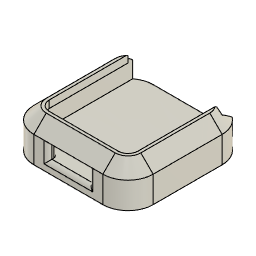
M8Q5883SlideMount (Autodesk Fusion 360 design; units mm, degrees)
Autodesk Fusion 360 part; units mm, degrees
sketch "M8QTop" plane through (0, 0, 0) normal (0, 0, 1) x (1, 0, 0) in component "M8Q"
  line L0 (-7.75, 7.925) -> (7.75, 7.925) construction
  line L1 (7.75, 7.925) -> (7.75, -7.925) construction
  line L2 (7.75, -7.925) -> (-7.75, -7.925) construction
  line L3 (-7.75, -7.925) -> (-7.75, 7.925) construction
  line L4 (0, 7.925) -> (0, -7.925) construction
  line L5 (-7.75, 0) -> (7.75, 0) construction
  line L6 (10, -10) -> (-10, -10) construction
  line L7 (0, 10) -> (0, -10) construction
  line L8 (-10, 10) -> (10, 10) construction
  line L9 (10, 10) -> (10, -10) construction
  line L10 (-10, -10) -> (-10, 10) construction
  line L11 (-10, 0) -> (10, 0) construction
  line L12 (-7, 10) -> (7, 10)
  line L13 (10, 7) -> (10, -7)
  line L14 (7, -10) -> (-7, -10)
  line L15 (-10, -7) -> (-10, 7)
  arc A0 (-7, 10) -> (-10, 7) centre (-7, 7) ccw
  arc A1 (10, 7) -> (7, 10) centre (7, 7) ccw
  arc A2 (7, -10) -> (10, -7) centre (7, -7) ccw
  arc A3 (-10, -7) -> (-7, -10) centre (-7, -7) ccw
  line L16 (-6, 7.925) -> (6, 7.925)
  line L17 (7.75, 6.175) -> (7.75, -6.175)
  line L18 (6, -7.925) -> (-6, -7.925)
  line L19 (-7.75, -6.175) -> (-7.75, 6.175)
  arc A4 (-6, 7.925) -> (-7.75, 6.175) centre (-6, 6.175) ccw
  arc A5 (7.75, 6.175) -> (6, 7.925) centre (6, 6.175) ccw
  arc A6 (6, -7.925) -> (7.75, -6.175) centre (6, -6.175) ccw
  arc A7 (-7.75, -6.175) -> (-6, -7.925) centre (-6, -6.175) ccw
  line L20 (-0.5, 9.134) -> (0.5, 9.134) construction
  line L21 (0.5, 9.134) -> (0, 10) construction
  line L22 (0, 10) -> (-0.5, 9.134) construction
  point P0 (-10, 10)
  point P1 (10, 10)
  point P2 (10, -10)
  point P3 (-7.75, 7.925)
  point P4 (7.75, 7.925)
  point P5 (7.75, -7.925)
  point P6 (0, 9.4226)
  dimension "d16" = 15.5
  dimension "d17" = 15.85
  dimension "d18" = 20
  dimension "d19" = 20
  dimension "d20" = 20
  dimension "d21" = 20
  dimension "d22" = 3
  dimension "d23" = 15.5
  dimension "d24" = 15.85
  dimension "d25" = 1.75
  dimension "d26" = 1
  constraint horizontal L0
  constraint vertical L1
  constraint horizontal L2
  constraint vertical L3
  constraint midpoint L0 L4.start
  constraint midpoint L2 L4.end
  constraint midpoint L3 L5.start
  constraint midpoint L1 L5.end
  constraint horizontal L8
  constraint vertical L9
  constraint horizontal L6
  constraint vertical L10
  constraint midpoint L7.start L8
  constraint midpoint L7.end L6
  constraint midpoint L11.start L10
  constraint midpoint L11.end L9
  constraint horizontal L12
  constraint vertical L13
  constraint horizontal L14
  constraint vertical L15
  constraint coincident P0 L12
  constraint coincident P0 L15
  constraint tangent L12 A0
  constraint tangent L15 A0
  constraint coincident P1 L12
  constraint coincident P1 L13
  constraint tangent L12 A1
  constraint tangent L13 A1
  constraint equal A0 A1
  constraint coincident P2 L13
  constraint coincident P2 L14
  constraint tangent L13 A2
  constraint tangent L14 A2
  constraint equal A0 A2
  constraint tangent L14 A3
  constraint tangent L15 A3
  constraint equal A0 A3
  constraint midpoint L7.start L12
  constraint midpoint origin L7
  constraint horizontal L16
  constraint vertical L17
  constraint horizontal L18
  constraint vertical L19
  constraint coincident P3 L16
  constraint coincident P3 L19
  constraint tangent L16 A4
  constraint tangent L19 A4
  constraint coincident P4 L16
  constraint coincident P4 L17
  constraint tangent L16 A5
  constraint tangent L17 A5
  constraint equal A4 A5
  constraint coincident P5 L17
  constraint coincident P5 L18
  constraint tangent L17 A6
  constraint tangent L18 A6
  constraint equal A4 A6
  constraint tangent L18 A7
  constraint tangent L19 A7
  constraint equal A4 A7
  constraint midpoint L4.start L16
  constraint midpoint origin L4
  constraint midpoint L12 L7.start
  measures "d16" distance of P3 P4
  measures "d17" distance of P4 P5
  measures "d18" distance of P0 P1
  measures "d19" distance of P1 P2
  measures "d20" distance of P0 P1
  measures "d21" distance of P1 P2
  measures "d22" radius of A0
  measures "d23" distance of P3 P4
  measures "d24" distance of P4 P5
  measures "d25" radius of A4
  measures "d26" distance of L20.start L20.end
sketch "M8QBottom" plane through (0, 0, 0) normal (0, 0, 1) x (1, 0, 0) in component "M8Q"
  line L0 (-4.15, 10) -> (4.15, 10)
  line L1 (4.15, 10) -> (4.15, 5.5)
  line L2 (4.15, 5.5) -> (-4.15, 5.5)
  line L3 (-4.15, 5.5) -> (-4.15, 10)
  line L4 (4.15, -5.5) -> (4.15, -10)
  line L5 (4.15, -10) -> (-4.15, -10)
  line L6 (-4.15, -10) -> (-4.15, -5.5)
  line L7 (-4.15, -5.5) -> (4.15, -5.5)
  line L8 (6.75, 0) -> (6.75, 2.75) construction
  line L9 (0, 0) -> (6.75, 0) construction
  circle A0 centre (6.75, 2.75) radius 2.375
  point P0 (0, 10)
  point P1 (0, -10)
  dimension "d30" = 8.3
  dimension "d31" = 4.5
  dimension "d37" = 4.5
  dimension "d39" = 8.3
  dimension "d40" = 2.75
  dimension "d41" = 6.75
  dimension "d42" = 4.75
  constraint horizontal L0
  constraint vertical L1
  constraint horizontal L2
  constraint vertical L3
  constraint horizontal L7
  constraint vertical L4
  constraint horizontal L5
  constraint vertical L6
  constraint midpoint L0 P0
  constraint midpoint L5 P1
  constraint vertical L8
  constraint horizontal L9
  constraint coincident L8.start L9.end
  constraint coincident L9.start origin
  constraint coincident L8.end A0.centre
  measures "d30" distance of L1.end L2.end
  measures "d31" distance of L0.end L1.end
  measures "d37" distance of L4.end L4.start
  measures "d39" distance of L4.start L6.end
  measures "d40" distance of L8.start L8.end
  measures "d41" distance of L9.start L8.start
  measures "d42" diameter of A0
extrude "Extrude Ports" add sketch "M8QBottom" along normal blind 3 contours L0 L1 L2 L3 | L4 L5 L6 L7 makes body 1 at (-1.3833, -7, 0) makes body 2 at (-1.3833, 8.5, 0) in component "M8Q"
extrude "M8Q" add sketch "M8QTop" along normal blind 1.25 from surface at 3 contours L12 L13 L14 L15 A0 A1 A2 A3 | L16 L17 L18 L19 A4 A5 A6 A7 bodies 1 2 in component "M8Q"
extrude "Extrude Battery" add sketch "M8QBottom" against normal blind 1.7 from surface at 3 contours A0 bodies 1 in component "M8Q"
extrude "Extrude4" add sketch "M8QTop" along normal blind 6.5 from surface at 4.25 contours L16 L17 L18 L19 A4 A5 A6 A7 bodies 1 in component "M8Q"
sketch "Profile" plane through (0, 0, 0) normal (0, 0, 1) x (1, 0, 0) in component "M8Q Mount"
  arc A0 (10, 7) -> (7, 10) centre (7, 7) ccw
  line L0 (10, 7) -> (10, -7)
  arc A1 (7, -10) -> (10, -7) centre (7, -7) ccw
  line L1 (7, -10) -> (-7, -10)
  arc A2 (-10, -7) -> (-7, -10) centre (-7, -7) ccw
  line L2 (-10, -7) -> (-10, 7)
  arc A3 (-7, 10) -> (-10, 7) centre (-7, 7) ccw
  line L3 (-7, 10) -> (7, 10)
  arc A4 (-7, 10.1) -> (-10.1, 7) centre (-7, 7) ccw
  line L4 (-10.1, -7) -> (-10.1, 7)
  arc A5 (-10.1, -7) -> (-7, -10.1) centre (-7, -7) ccw
  line L5 (7, -10.1) -> (-7, -10.1)
  arc A6 (7, -10.1) -> (10.1, -7) centre (7, -7) ccw
  line L6 (10.1, 7) -> (10.1, -7)
  arc A7 (10.1, 7) -> (7, 10.1) centre (7, 7) ccw
  line L7 (-7, 10.1) -> (7, 10.1)
  arc A8 (-7, 12.1) -> (-12.1, 7) centre (-7, 7) ccw
  line L8 (-12.1, -7) -> (-12.1, 7)
  arc A9 (-12.1, -7) -> (-7, -12.1) centre (-7, -7) ccw
  line L9 (7, -12.1) -> (-7, -12.1)
  arc A10 (7, -12.1) -> (12.1, -7) centre (7, -7) ccw
  line L10 (12.1, 7) -> (12.1, -7)
  arc A11 (12.1, 7) -> (7, 12.1) centre (7, 7) ccw
  line L11 (-7, 12.1) -> (7, 12.1)
  arc A12 (-7, 9) -> (-9, 7) centre (-7, 7) ccw
  line L12 (-9, -7) -> (-9, 7)
  arc A13 (-9, -7) -> (-7, -9) centre (-7, -7) ccw
  line L13 (7, -9) -> (-7, -9)
  arc A14 (7, -9) -> (9, -7) centre (7, -7) ccw
  line L14 (9, 7) -> (9, -7)
  arc A15 (9, 7) -> (7, 9) centre (7, 7) ccw
  line L15 (-7, 9) -> (7, 9)
  dimension "d57" = 0.1
  dimension "d58" = 2.1
  dimension "d60" = -1
sketch "Cuts" plane through (0, 0, 0) normal (0, 0, 1) x (1, 0, 0) in component "M8Q Mount"
  arc A0 (-7, 9) -> (-9, 7) centre (-7, 7) ccw
  line L0 (-7, 9) -> (7, 9)
  arc A1 (9, 7) -> (7, 9) centre (7, 7) ccw
  line L1 (9, 7) -> (9, -7)
  arc A2 (7, -9) -> (9, -7) centre (7, -7) ccw
  line L2 (7, -9) -> (-7, -9)
  arc A3 (-9, -7) -> (-7, -9) centre (-7, -7) ccw
  line L3 (-9, -7) -> (-9, 7)
  arc A4 (12.1, 7) -> (7, 12.1) centre (7, 7) ccw
  line L4 (12.1, 7) -> (12.1, -7)
  arc A5 (7, -12.1) -> (12.1, -7) centre (7, -7) ccw
  line L5 (7, -12.1) -> (-7, -12.1)
  arc A6 (-12.1, -7) -> (-7, -12.1) centre (-7, -7) ccw
  line L6 (-12.1, -7) -> (-12.1, 7)
  arc A7 (-7, 12.1) -> (-12.1, 7) centre (-7, 7) ccw
  line L7 (-7, 12.1) -> (7, 12.1)
  line L8 (4.15, -5.5) -> (4.15, -10)
  line L9 (4.15, -10) -> (-4.15, -10)
  line L10 (-4.15, -10) -> (-4.15, -5.5)
  line L11 (-4.15, -5.5) -> (4.15, -5.5)
  line L12 (-10.1, 7) -> (10.1, 7)
  line L13 (10.1, 7) -> (10.1, 12.1)
  line L14 (10.1, 12.1) -> (-10.1, 12.1)
  line L15 (-10.1, 12.1) -> (-10.1, 7)
  line L16 (-4.15, -5.5) -> (4.15, -5.5)
  line L17 (4.15, -5.5) -> (4.15, -12.1)
  line L18 (4.15, -12.1) -> (-4.15, -12.1)
  line L19 (-4.15, -12.1) -> (-4.15, -5.5)
  line L20 (-10.1, -7) -> (-10.1, 7)
  arc A8 (-10.1, -7) -> (-7, -10.1) centre (-7, -7) ccw
  line L21 (7, -10.1) -> (-7, -10.1)
  arc A9 (7, -10.1) -> (10.1, -7) centre (7, -7) ccw
  line L22 (10.1, 7) -> (10.1, -7)
  arc A10 (10.1, 7) -> (7, 10.1) centre (7, 7) ccw
  line L23 (-7, 10.1) -> (7, 10.1)
  arc A11 (-7, 10.1) -> (-10.1, 7) centre (-7, 7) ccw
  line L24 (-9, 0) -> (9, 0)
  line L25 (9, 0) -> (9, 12.1)
  line L26 (9, 12.1) -> (-9, 12.1)
  line L27 (-9, 12.1) -> (-9, 0)
  line L28 (-10.1, 12.1) -> (10.1, 12.1)
  line L29 (10.1, 12.1) -> (10.1, 9)
  line L30 (10.1, 9) -> (-10.1, 9)
  line L31 (-10.1, 9) -> (-10.1, 12.1)
  point P0 (-10.1, 7)
  constraint perpendicular L12 L13
  constraint parallel L12 L14
  constraint parallel L13 L15
  constraint perpendicular L1 L12
  constraint collinear L7 L14
  constraint perpendicular L16 L17
  constraint parallel L16 L18
  constraint parallel L17 L19
  constraint coincident L8.start L11.end
  constraint perpendicular L8 L16
  constraint coincident L10.end L11.start
  constraint collinear L5 L18
  constraint collinear L13 L22
  constraint collinear L15 L20
  constraint perpendicular L24 L25
  constraint parallel L25 L27
  constraint midpoint L1 L24.end
  constraint perpendicular L1 L24
  constraint midpoint L3 L24.start
  constraint collinear L14 L26
  constraint coincident P0 L12.start
  constraint perpendicular L28 L29
  constraint parallel L28 L30
  constraint parallel L29 L31
  constraint collinear L0 L30
extrude "Extude Base" add sketch "Profile" against normal blind 2 separate body contours A0 L0 A1 L1 A2 L2 A3 L3 | A4 L4 A5 L5 A6 L6 A7 L7 | A8 L8 A9 L9 A10 L10 A11 L11 | A12 L12 A13 L13 A14 L14 A15 L15 makes body 3 in component "M8Q Mount"
extrude "Extude Walls" add sketch "Profile" along normal blind 5.85 contours A0 L0 A1 L1 A2 L2 A3 L3 | A4 L4 A5 L5 A6 L6 A7 L7 | A8 L8 A9 L9 A10 L10 A11 L11 bodies 3 in component "M8Q Mount"
extrude "Cut Inner" cut sketch "Profile" along normal blind 4.35 contours A0 L0 A1 L1 A2 L2 A3 L3 | A4 L4 A5 L5 A6 L6 A7 L7 bodies 3 in component "M8Q Mount"
chamfer "Chamfer Walls" distance 2.5 angle 45 8 edges at (12.1, 0, 5.85) (10.6062, 10.6062, 5.85) (0, 12.1, 5.85) (-10.6062, 10.6062, 5.85) (-12.1, 0, 5.85) (-10.6062, -10.6062, 5.85) (0, -12.1, 5.85) (10.6062, -10.6062, 5.85) on bodies 3 in component "M8Q Mount"
extrude "Cut Bottom Port" cut sketch "Cuts" along normal blind 3 contours L2 L8 L10 L11 L16 L17 L19 | L2 L8 L9 L10 L17 L19 | L5 L17 L18 L19 L21 | L9 L17 L19 L21 bodies 3 in component "M8Q Mount"
extrude "Cut Top" cut sketch "Cuts" along normal blind 4.35 contours A0 L0 A1 L12 L30 | L0 A10 L23 A11 L25 L27 L30 | A0 L27 L30 | L12 A11 L27 L30 | A1 L25 L30 | A11 L27 L30 | L15 A11 L30 | L12 A10 L25 L30 | A10 L25 L30 | A4 A7 L7 L14 A10 L23 A11 L25 L26 L27 L28 | A7 L15 A11 L27 L30 L31 | L13 A10 L30 | A4 L13 A10 L25 L29 L30 | A7 L14 L26 L27 L28 | A7 L14 L15 L27 L28 L31 | A4 L13 L14 L25 L28 L29 | A4 L14 L25 L26 L28 bodies 3 in component "M8Q Mount"
extrude "Extrude6" cut sketch "Cuts" along normal through all contours A0 L0 A1 L12 L30 | L0 A10 L23 A11 L25 L27 L30 | A0 L27 L30 | A1 L25 L30 | A11 L27 L30 | A10 L25 L30 | A4 A7 L7 L14 A10 L23 A11 L25 L26 L27 L28 | A7 L15 A11 L27 L30 L31 | A4 L13 A10 L25 L29 L30 | A7 L14 L26 L27 L28 | A7 L14 L15 L27 L28 L31 | A4 L13 L14 L25 L28 L29 | A4 L14 L25 L26 L28 bodies 3 in component "M8Q Mount"
fillet "Chamfer Port" radius 0.8 7 edges at (0, -12.1, 0) (-4.15, -12.1, 1.5) (0, -12.1, 3) (4.15, -12.1, 1.5) (4.15, -10.1, 1.5) (0, -10.1, 3) (-4.15, -10.1, 1.5) on bodies 3 in component "M8Q Mount"
component "M8Q" placed x (1, 0, 0) y (0, 1, 0) z (0, 0, 1) at (0, 0, 0)
component "M8Q Mount" placed x (1, 0, 0) y (0, 1, 0) z (0, 0, 1) at (0, 0, 0)
component "Joiner" placed x (1, 0, 0) y (0, 1, 0) z (0, 0, 1) at (0, 0, 0)
equation "M8QBoardSide = 20 mm" comment "Sides of the M8Q circuit board"
equation "M8QBoardHeight = 1.25 mm" comment "Height (thickness) of M8Q circuit board."
equation "M8QPortWidth = 8.3 mm" comment "Width of the M8Q connector ports."
equation "M8QPortHeight = 3 mm" comment "Height of the M8Q connector ports."
equation "M8QBatteryDiameter = 4.75 mm" comment "Diameter of the hot start battery."
equation "M8QBatteryHeight = 1.7 mm" comment "Height of the hot start battery"
equation "M8QBatteryMidOffset = 2.75 mm" comment "Offset from board middle to battery."
equation "M8QBatteryCenterOffset = 6.75 mm" comment "Offset from board center to batery center"
equation "M8QAntennaWidth = 15.5 mm" comment "Width of the antenna and board."
equation "M8QAntennaLength = 15.85 mm" comment "Length of the antenna and board."
equation "M8QAntennaHeight = 6.5 mm" comment "Height of the antenna and board."
equation "M8QHeight = M8QPortHeight + M8QBoardHeight + M8QAntennaHeight" comment "Total height of the M8Q module"
equation "M8QPortBoardHeight = M8QPortHeight + M8QBoardHeight" comment "Height of port and board."
equation "M8QBoardFilet = 3 mm" comment "Radius of board filet."
equation "M8QAntennaFilet = 1.75 mm" comment "Radius of antenna filet."
equation "d16 = M8QAntennaWidth"
equation "d17 = M8QAntennaLength"
equation "d18 = M8QBoardSide"
equation "d19 = M8QBoardSide"
equation "d20 = M8QBoardSide"
equation "d21 = M8QBoardSide"
equation "d22 = M8QBoardFilet"
equation "d23 = M8QAntennaWidth"
equation "d24 = M8QAntennaLength"
equation "d25 = M8QAntennaFilet"
equation "M8QPortLength = 4.5 mm" comment "Length of the connector ports"
equation "d30 = M8QPortWidth"
equation "d31 = M8QPortLength"
equation "d37 = M8QPortLength"
equation "d39 = M8QPortWidth"
equation "d40 = M8QBatteryMidOffset"
equation "d41 = M8QBatteryCenterOffset"
equation "d42 = M8QBatteryDiameter"
equation "d43 = M8QPortHeight"
equation "d45 = M8QPortHeight"
equation "d46 = M8QBoardHeight"
equation "d48 = M8QPortHeight"
equation "d49 = -M8QBatteryHeight"
equation "d51 = M8QPortHeight + M8QBoardHeight"
equation "d52 = M8QAntennaHeight"
equation "M8QMountGap = 0.1 mm" comment "Inner gap between module and mount"
equation "M8QMountThickness = 2 mm" comment "Thickness of the mount walls."
equation "M8QMountChamfer = 2.5 mm" comment "Radius of the mount filet"
equation "d57 = M8QMountGap"
equation "d58 = M8QMountGap + M8QMountThickness"
equation "M8QMountOverlap = 1 mm" comment "How much the mount overlaps the board."
equation "d60 = -M8QMountOverlap"
equation "M8QMountBaseHeight = 2 mm" comment "Height of the mount base."
equation "M8QMountTopHeight = 1.5 mm" comment "Height of the mount top."
equation "d63 = -M8QMountBaseHeight"
equation "d65 = M8QPortBoardHeight + M8QMountGap + M8QMountTopHeight"
equation "d67 = M8QPortBoardHeight + M8QMountGap"
equation "d69 = M8QMountChamfer"
equation "d71 = M8QPortHeight"
equation "d73 = M8QPortBoardHeight + M8QMountGap"
equation "d77 = MQ8MountPortChamfer"
equation "MQ8MountPortChamfer = 0.8 mm" comment "Radius of the port chamfer"
named bodies: "M8Q", "Port Back", "M8Q Mount"
